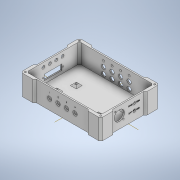
# Autodesk Inventor part: Case
Saved by Autodesk Inventor 2021.1 (Build 251245000, 245)
## iProperties
Created: 2020-06-02
Part Number: Case
Material: Generic
Document SubType Name: Modeling
Designer: Alex
Density: 1 g/cm^3
Appearance: Default
Author: Alex
Autodesk Inventor part; units mm, degrees
note: some values were not read from the file. Chosen so that the rebuilt part matches the saved one: direction of "Hole1"; direction of "Hole2"; direction of "Hole4"; direction of "Hole6"; direction of "Hole7".
(part 1 of 2)
ref_plane "YZ Plane" through (0, 0, 0) normal (1, 0, 0) x (0, 1, 0)
ref_plane "XZ Plane" through (0, 0, 0) normal (0, 1, 0) x (-1, 0, 0)
ref_plane "XY Plane" through (0, 0, 0) normal (0, 0, 1) x (1, 0, 0)
sketch "Sketch1" plane through (0, 0, 0) normal (0, 1, 0) x (-1, 0, 0)
  line L0 (61, -65) -> (-61, -65)
  line L1 (-61, -65) -> (-65, -69)
  line L2 (-65, -69) -> (-90, -69)
  line L3 (-90, -69) -> (-94, -65)
  line L4 (-94, -65) -> (-94, -40)
  line L5 (-94, -40) -> (-90, -36)
  line L6 (-90, -36) -> (-90, 36)
  line L7 (-90, 36) -> (-94, 40)
  line L8 (-94, 40) -> (-94, 65)
  line L9 (-94, 65) -> (-90, 69)
  line L10 (-90, 69) -> (-65, 69)
  line L11 (-65, 69) -> (-61, 65)
  line L12 (-61, 65) -> (61, 65)
  line L13 (61, 65) -> (65, 69)
  line L14 (65, 69) -> (90, 69)
  line L15 (90, 69) -> (94, 65)
  line L16 (94, 65) -> (94, 40)
  line L17 (94, 40) -> (90, 36)
  line L18 (90, 36) -> (90, -36)
  line L19 (90, -36) -> (94, -40)
  line L20 (94, -40) -> (94, -65)
  line L21 (94, -65) -> (90, -69)
  line L22 (90, -69) -> (65, -69)
  line L23 (65, -69) -> (61, -65)
  point P0 (0, 0)
  point P1 (0, -65)
  point P2 (0, 65)
  point P3 (90, 0)
  point P4 (-90, 0)
  dimension "d0" = 135
  dimension "d1" = 130
  dimension "d2" = 180
  dimension "d3" = 4
  dimension "d4" = 25
  constraints: 48 end point, 9 equal length, 9 parallel, 9 perpendicular, 6 point on line, 4 midpoint, 3 collinear, 3 horizontal alignment, 3 vertical alignment, 1 horizontal
  measures "d0" angle of L0 L23
  measures "d1" distance between parallel lines of L12 L0
  measures "d2" distance between parallel lines of L6 L18
  measures "d3" distance between parallel lines of L0 L2
  measures "d4" distance of L1.end L2.end
extrude "Extrusion1" add sketch "Sketch1" along normal blind 3
sketch "Sketch2" plane through (0, 3, 0) normal (0, 1, 0) x (1, 0, 0)
  line L0 (94, 65) -> (90, 69) projected
  line L1 (90, 69) -> (65, 69) projected
  line L2 (65, 69) -> (61, 65) projected
  line L3 (61, 65) -> (-61, 65) projected
  line L4 (-61, 65) -> (-65, 69) projected
  line L5 (-65, 69) -> (-90, 69) projected
  line L6 (-90, 69) -> (-94, 65) projected
  line L7 (-94, 65) -> (-94, 40) projected
  line L8 (-94, 40) -> (-90, 36) projected
  line L9 (-90, 36) -> (-90, -36) projected
  line L10 (-90, -36) -> (-94, -40) projected
  line L11 (-94, -40) -> (-94, -65) projected
  line L12 (-94, -65) -> (-90, -69) projected
  line L13 (-90, -69) -> (-65, -69) projected
  line L14 (-65, -69) -> (-61, -65) projected
  line L15 (-61, -65) -> (61, -65) projected
  line L16 (61, -65) -> (65, -69) projected
  line L17 (65, -69) -> (90, -69) projected
  line L18 (90, -69) -> (94, -65) projected
  line L19 (94, -65) -> (94, -40) projected
  line L20 (94, -40) -> (90, -36) projected
  line L21 (90, -36) -> (90, 36) projected
  line L22 (90, 36) -> (94, 40) projected
  line L23 (94, 40) -> (94, 65) projected
  line L24 (-62.2426, 62) -> (62.2426, 62)
  line L25 (62.2426, 62) -> (66.2426, 66) construction
  line L26 (66.2426, 66) -> (88.7574, 66) construction
  line L27 (88.7574, 66) -> (91, 63.7574) construction
  line L28 (91, 63.7574) -> (91, 41.2426) construction
  line L29 (91, 41.2426) -> (87, 37.2426) construction
  line L30 (87, 37.2426) -> (87, -37.2426)
  line L31 (87, -37.2426) -> (91, -41.2426) construction
  line L32 (91, -41.2426) -> (91, -63.7574) construction
  line L33 (91, -63.7574) -> (88.7574, -66) construction
  line L34 (88.7574, -66) -> (66.2426, -66) construction
  line L35 (66.2426, -66) -> (62.2426, -62) construction
  line L36 (62.2426, -62) -> (-62.2426, -62)
  line L37 (-62.2426, -62) -> (-66.2426, -66) construction
  line L38 (-66.2426, -66) -> (-88.7574, -66) construction
  line L39 (-88.7574, -66) -> (-91, -63.7574) construction
  line L40 (-91, -63.7574) -> (-91, -41.2426) construction
  line L41 (-91, -41.2426) -> (-87, -37.2426) construction
  line L42 (-87, -37.2426) -> (-87, 37.2426)
  line L43 (-87, 37.2426) -> (-91, 41.2426) construction
  line L44 (-91, 41.2426) -> (-91, 63.7574) construction
  line L45 (-91, 63.7574) -> (-88.7574, 66) construction
  line L46 (-88.7574, 66) -> (-66.2426, 66) construction
  line L47 (-66.2426, 66) -> (-62.2426, 62) construction
  line L48 (-62.2426, 62) -> (-83, 62)
  line L49 (-87, 58) -> (-87, 37.2426)
  line L50 (-87, -37.2426) -> (-87, -58)
  line L51 (-83, -62) -> (-62.2426, -62)
  line L52 (62.2426, -62) -> (83, -62)
  line L53 (87, -58) -> (87, -37.2426)
  line L54 (62.2426, 62) -> (83, 62)
  line L55 (87, 58) -> (87, 37.2426)
  line L56 (-87, 58) -> (-83, 62)
  line L57 (-87, -58) -> (-83, -62)
  line L58 (83, -62) -> (87, -58)
  line L59 (87, 58) -> (83, 62)
  point P0 (0, 0)
  point P1 (-87, 62)
  point P2 (-87, -62)
  point P3 (87, -62)
  point P4 (87, 62)
  dimension "d7" = 3
  dimension "d8" = 4
  dimension "d9" = 4
  dimension "d10" = 4
  dimension "d11" = 4
  dimension "d12" = 4
  dimension "d13" = 4
  dimension "d14" = 4
  dimension "d15" = 4
  constraints: 72 end point, 9 point on line, 4 horizontal, 2 perpendicular, 1 vertical, 23 other
  measures "d7" distance between parallel lines of L3 L24
  measures "d8" distance of L49.start point (-87, 62)
  measures "d9" distance of L48.end point (-87, 62)
  measures "d10" distance of L50.end point (-87, -62)
  measures "d11" distance of L51.start point (-87, -62)
  measures "d12" distance of L52.end point (87, -62)
  measures "d13" distance of L53.start point (87, -62)
  measures "d14" distance of L55.start point (87, 62)
  measures "d15" distance of L54.end point (87, 62)
extrude "Extrusion2" add sketch "Sketch2" along normal blind 45
sketch "Sketch3" plane through (0, 3, 0) normal (0, 1, 0) x (1, 0, 0)
  line L0 (60.58, -23.875) -> (-60.58, -23.875) construction
  line L1 (-60.58, -23.875) -> (-60.58, 23.875) construction
  line L2 (-60.58, 23.875) -> (60.58, 23.875) construction
  line L3 (60.58, 23.875) -> (60.58, -23.875) construction
  line L4 (60.58, -23.875) -> (-60.58, 23.875) construction
  line L5 (-60.58, -23.875) -> (60.58, 23.875) construction
  line L6 (-49.356, 16.969) -> (-43.356, 16.969)
  line L7 (-43.356, 16.969) -> (-43.356, 10.969)
  line L8 (-43.356, 10.969) -> (-49.356, 10.969)
  line L9 (-49.356, 10.969) -> (-49.356, 16.969)
  line L10 (-49.356, 16.969) -> (-43.356, 10.969) construction
  line L11 (-43.356, 16.969) -> (-49.356, 10.969) construction
  line L12 (-60.278, -23.575) -> (-54.278, -23.575)
  line L13 (-54.278, -23.575) -> (-54.278, -17.575)
  line L14 (-54.278, -17.575) -> (-60.278, -17.575)
  line L15 (-60.278, -17.575) -> (-60.278, -23.575)
  line L16 (-60.278, -23.575) -> (-54.278, -17.575) construction
  line L17 (-54.278, -23.575) -> (-60.278, -17.575) construction
  line L18 (37.004, -17.575) -> (43.004, -17.575)
  line L19 (43.004, -17.575) -> (43.004, -23.575)
  line L20 (43.004, -23.575) -> (37.004, -23.575)
  line L21 (37.004, -23.575) -> (37.004, -17.575)
  line L22 (37.004, -17.575) -> (43.004, -23.575) construction
  line L23 (43.004, -17.575) -> (37.004, -23.575) construction
  line L24 (54.276, 23.573) -> (60.276, 23.573)
  line L25 (60.276, 23.573) -> (60.276, 17.573)
  line L26 (60.276, 17.573) -> (54.276, 17.573)
  line L27 (54.276, 17.573) -> (54.276, 23.573)
  line L28 (54.276, 23.573) -> (60.276, 17.573) construction
  line L29 (60.276, 23.573) -> (54.276, 17.573) construction
  point P0 (0, 0)
  point P1 (-46.356, 13.969)
  point P2 (-57.278, -20.575)
  point P3 (40.004, -20.575)
  point P4 (57.276, 20.573)
  dimension "d18" = 121.16
  dimension "d19" = 47.75
  dimension "d20" = 9.906
  dimension "d21" = 14.224
  dimension "d28" = 6
  dimension "d188" = 3.302
  dimension "d189" = 44.45
  dimension "d190" = 117.856
  dimension "d191" = 3.302
  dimension "d192" = 100.584
  dimension "d193" = 44.45
  constraints: 60 end point, 10 midpoint, 10 parallel, 6 equal length, 5 horizontal, 5 perpendicular, 1 point on line
  measures "d18" distance of L1.end L2.end
  measures "d19" distance of L2.end L0.start
  measures "d20" distance from line of point (-46.356, 13.969) L2
  measures "d21" distance from line of point (-46.356, 13.969) L1
  measures "d28" distance of L6.end L7.end
  measures "d188" distance from line of point (-57.278, -20.575) L1
  measures "d189" distance from line of point (-57.278, -20.575) L2
  measures "d190" distance from line of point (57.276, 20.573) L1
  measures "d191" distance from line of point (57.276, 20.573) L2
  measures "d192" distance from line of point (40.004, -20.575) L1
  measures "d193" distance from line of point (40.004, -20.575) L2
extrude "Extrusion3" add sketch "Sketch3" along normal blind 4
chamfer "Chamfer1" distance 4 angle 45 16 edges at (40.004, 3, 23.575) (43.004, 3, 20.575) (57.276, 3, -17.573) (60.276, 3, -20.573) (37.004, 3, 20.575) (54.276, 3, -20.573) (40.004, 3, 17.575) (57.276, 3, -23.573) (-57.278, 3, 17.575) (-60.278, 3, 20.575) (-46.356, 3, -16.969) (-49.356, 3, -13.969) (-57.278, 3, 23.575) (-54.278, 3, 20.575) (-46.356, 3, -10.969) (-43.356, 3, -13.969)
sketch "Sketch4" plane through (-61, 0, 65) normal (0, 0, 1) x (1, 0, 0)
  line L0 (0, 0) -> (122, 0) construction
  line L1 (122, 0) -> (122, 48) construction
  line L2 (0, 48) -> (122, 48) construction
  line L3 (0, 0) -> (0, 48) construction
  line L4 (0, 0) -> (0, 48) construction
  line L5 (0, 48) -> (122, 48) construction
  line L6 (61, 48) -> (61, 0) construction
  point P0 (31, 24)
  point P1 (51, 24)
  point P2 (71, 24)
  point P3 (91, 24)
  point P4 (0, 24)
  point P5 (0, 24)
  dimension "d36" = 20
  constraints: 3 midpoint, 2 end point, 1 horizontal, 1 horizontal alignment, 1 perpendicular, 1 symmetric about line, 3 other
  measures "d36" distance of point (31, 24) point (51, 24)
hole "Hole1" at (-30, 24, 65) at (-10, 24, 65) at (10, 24, 65) at (30, 24, 65) direction (0, 0, -1) diameter 10.317 depth 3 clearance for "Hex Head Bolt" size "3/8" standard "Ansi Unified Screw Threads"
sketch "Sketch5" plane through (61, 0, -65) normal (0, 0, -1) x (-1, 0, 0)
  line L0 (0, 0) -> (122, 0) construction
  line L1 (122, 0) -> (122, 48) construction
  line L2 (0, 48) -> (122, 48) construction
  line L3 (0, 0) -> (0, 48) construction
  line L4 (0, 0) -> (0, 48) construction
  line L5 (122, 48) -> (0, 48) construction
  line L6 (61, 48) -> (61, 0) construction
  point P0 (31, 10)
  point P1 (51, 10)
  point P2 (71, 10)
  point P3 (91, 10)
  point P4 (31, 25)
  point P5 (51, 25)
  point P6 (71, 25)
  point P7 (91, 25)
  dimension "d50" = 20
  dimension "d53" = 15
  dimension "d115" = 10
  constraints: 2 end point, 2 vertical, 1 horizontal, 1 midpoint, 1 symmetric about line, 7 other
  measures "d50" distance of point (31, 10) point (51, 10)
  measures "d53" distance of point (31, 10) point (31, 25)
  measures "d115" distance from line of L0 point (31, 10)
hole "Hole2" at (30, 10, -65) at (10, 10, -65) at (-10, 10, -65) at (-30, 10, -65) at (30, 25, -65) at (10, 25, -65) at (-10, 25, -65) at (-30, 25, -65) direction (0, 0, 1) diameter 10.317 depth 3 clearance for "Hex Head Bolt" size "3/8" standard "Ansi Unified Screw Threads"
sketch "Sketch6" plane through (0, 7, 0) normal (0, 1, 0) x (1, 0, 0)
  line L0 (43.004, -17.575) -> (37.004, -17.575) construction
  line L1 (37.004, -17.575) -> (37.004, -23.575) construction
  line L2 (37.004, -23.575) -> (43.004, -23.575) construction
  line L3 (43.004, -23.575) -> (43.004, -17.575) construction
  line L4 (60.276, 23.573) -> (54.276, 23.573) construction
  line L5 (54.276, 23.573) -> (54.276, 17.573) construction
  line L6 (54.276, 17.573) -> (60.276, 17.573) construction
  line L7 (60.276, 17.573) -> (60.276, 23.573) construction
  line L8 (-49.356, 10.969) -> (-43.356, 10.969) construction
  line L9 (-43.356, 10.969) -> (-43.356, 16.969) construction
  line L10 (-43.356, 16.969) -> (-49.356, 16.969) construction
  line L11 (-49.356, 16.969) -> (-49.356, 10.969) construction
  line L12 (-60.278, -17.575) -> (-60.278, -23.575) construction
  line L13 (-60.278, -23.575) -> (-54.278, -23.575) construction
  line L14 (-54.278, -23.575) -> (-54.278, -17.575) construction
  line L15 (-54.278, -17.575) -> (-60.278, -17.575) construction
  point P0 (0, 0)
  point P1 (40.004, -20.575)
  point P2 (57.276, 20.573)
  point P3 (-46.356, 13.969)
  point P4 (-57.278, -20.575)
  point P5 (37.004, -20.575)
  point P6 (-60.278, -20.575)
  point P7 (-49.356, 13.969)
  point P8 (54.276, 20.573)
  point P9 (40.004, -17.575)
  point P10 (57.276, 23.573)
  point P11 (-46.356, 16.969)
  point P12 (-57.278, -17.575)
  constraints: 8 midpoint, 4 horizontal alignment, 4 vertical alignment
hole "Hole3" at (40.004, 7, 20.575) at (57.276, 7, -20.573) at (-46.356, 7, -13.969) at (-57.278, 7, 20.575) direction (0, -1, 0) diameter 4 depth 5
sketch "Sketch7" plane through (-90, 0, -36) normal (-1, 0, 0) x (0, 0, 1)
  line L0 (57, 10) -> (15, 10)
  line L1 (15, 10) -> (15, 23)
  line L2 (15, 23) -> (57, 23)
  line L3 (57, 23) -> (57, 10)
  line L4 (57, 10) -> (15, 23) construction
  line L5 (15, 10) -> (57, 23) construction
  line L6 (0, 0) -> (72, 0) construction
  line L7 (72, 0) -> (72, 48) construction
  line L8 (0, 48) -> (72, 48) construction
  line L9 (0, 0) -> (0, 48) construction
  point P0 (36, 0)
  point P1 (36, 16.5)
  point P2 (36, 48)
  point P3 (36, 16.5)
  point P4 (15, 16.5)
  point P5 (0, 24)
  dimension "d70" = 42
  dimension "d71" = 13
  dimension "d131" = 10
  constraints: 12 end point, 6 midpoint, 2 parallel, 1 horizontal, 1 perpendicular, 1 vertical alignment
  measures "d70" distance of L1.end L2.end
  measures "d71" distance of L2.end L0.start
  measures "d131" distance between parallel lines of L6 L0
extrude "Extrusion4" cut sketch "Sketch7" against normal up to surface (3 mm away)
sketch "Sketch8" plane through (-90, 0, -36) normal (-1, 0, 0) x (0, 0, 1)
  line L0 (9.5, 23) -> (62.5, 23) construction
  line L1 (62.5, 23) -> (62.5, 10) construction
  line L2 (62.5, 10) -> (9.5, 10) construction
  line L3 (9.5, 10) -> (9.5, 23) construction
  line L4 (15, 23) -> (57, 23) construction
  line L5 (57, 23) -> (57, 10) construction
  line L6 (57, 10) -> (15, 10) construction
  line L7 (15, 10) -> (15, 23) construction
  line L8 (0, 0) -> (72, 0) construction
  line L9 (72, 0) -> (72, 48) construction
  line L10 (0, 48) -> (72, 48) construction
  line L11 (0, 0) -> (0, 48) construction
  point P0 (36, 0)
  point P1 (36, 23)
  point P2 (36, 23)
  point P3 (15, 16.5)
  point P4 (9.5, 16.5)
  point P5 (12.5, 16.5)
  point P6 (59.5, 16.5)
  point P7 (57, 16.5)
  dimension "d75" = 53
  dimension "d76" = 3
  dimension "d77" = 3
  constraints: 8 end point, 5 midpoint, 3 horizontal alignment, 2 parallel, 1 coincident, 1 collinear, 1 horizontal, 1 perpendicular
  measures "d75" distance between parallel lines of L3 L1
  measures "d76" distance from line of L3 point (12.5, 16.5)
  measures "d77" distance from line of L1 point (59.5, 16.5)
hole "Hole4" at (-90, 16.5, -23.5) at (-90, 16.5, 23.5) direction (1, 0, 0) diameter 3 depth 3
sketch "Sketch9" plane through (90, 0, 36) normal (1, 0, 0) x (0, 0, -1)
  circle A0 centre (15, 27.5) radius 12
  circle A1 centre (5.5, 39.5) radius 1.75
  circle A2 centre (24.5, 15.5) radius 1.75
  line L0 (28, 12) -> (2, 12) construction
  line L1 (2, 12) -> (2, 43) construction
  line L2 (2, 43) -> (28, 43) construction
  line L3 (28, 43) -> (28, 12) construction
  line L4 (28, 12) -> (2, 43) construction
  line L5 (2, 12) -> (28, 43) construction
  line L6 (0, 0) -> (72, 0) construction
  line L7 (72, 0) -> (72, 48) construction
  line L8 (0, 48) -> (72, 48) construction
  line L9 (0, 0) -> (0, 48) construction
  circle A3 centre (50, 35) radius 3.25
  circle A4 centre (50, 20) radius 3.25
  line L10 (28, 43) -> (72, 43) construction
  line L11 (50, 35) -> (50, 20) construction
  point P0 (36, 0)
  point P1 (2, 27.5)
  point P2 (0, 24)
  point P3 (50, 43)
  point P4 (28, 27.5)
  point P5 (50, 27.5)
  dimension "d85" = 19
  dimension "d86" = 24
  dimension "d87" = 24
  dimension "d88" = 9.5
  dimension "d89" = 12
  dimension "d90" = 3.5
  dimension "d91" = 26
  dimension "d92" = 31
  dimension "d93" = 2
  dimension "d94" = 6.5
  dimension "d95" = 15
  dimension "d194" = 5
  constraints: 16 end point, 7 midpoint, 5 centre point, 2 equal radius, 2 parallel, 2 perpendicular, 2 vertical alignment, 1 horizontal, 1 horizontal alignment, 1 point on line, 1 vertical
  measures "d85" horizontal distance of A2.centre A1.centre
  measures "d86" vertical distance of A2.centre A1.centre
  measures "d87" diameter of A0
  measures "d88" horizontal distance of A0.centre A1.centre
  measures "d89" vertical distance of A0.centre A1.centre
  measures "d90" diameter of A1
  measures "d91" distance of L1.end L2.end
  measures "d92" distance of L2.end L0.start
  measures "d93" distance between parallel lines of L9 L1
  measures "d94" diameter of A3
  measures "d95" distance of L11.start L11.end
  measures "d194" distance between parallel lines of L2 L8
extrude "Extrusion5" cut sketch "Sketch9" against normal up to surface (3 mm away)
sketch "Sketch11" plane through (61, 0, -65) normal (0, 0, -1) x (-1, 0, 0)
  line L0 (-4, 0) -> (0, 0) construction
  line L1 (0, 0) -> (0, 48) construction
  line L2 (-4, 48) -> (0, 48) construction
  line L3 (-4, 0) -> (-4, 48) construction
  circle A0 centre (71, 25) radius 5.1585 construction
  circle A1 centre (31, 25) radius 5.1585 construction
  circle A2 centre (71, 10) radius 5.1585 construction
  circle A3 centre (31, 10) radius 5.1585 construction
  circle A4 centre (51, 10) radius 5.1585 construction
  circle A5 centre (91, 10) radius 5.1585 construction
  circle A6 centre (51, 25) radius 5.1585 construction
  circle A7 centre (91, 25) radius 5.1585 construction
  line L4 (0, 0) -> (122, 0) construction
  line L5 (122, 0) -> (122, 48) construction
  line L6 (0, 48) -> (122, 48) construction
  line L7 (0, 0) -> (0, 48) construction
  point P0 (61, 0)
  point P1 (31, 37.5)
  point P2 (51, 37.5)
  point P3 (71, 37.5)
  point P4 (91, 37.5)
  dimension "d118" = 20
  dimension "d147" = 12.5
  constraints: 1 horizontal, 1 vertical alignment, 3 other
  measures "d118" distance of point (31, 37.5) point (51, 37.5)
  measures "d147" distance of A1.centre point (31, 37.5)
hole "Hole6" at (30, 37.5, -65) at (10, 37.5, -65) at (-10, 37.5, -65) at (-30, 37.5, -65) direction (0, 0, 1) diameter 5 depth 3
sketch "Sketch12" plane through (-90, 0, -36) normal (-1, 0, 0) x (0, 0, 1)
  circle A0 centre (12.5, 16.5) radius 1.5 construction
  circle A1 centre (59.5, 16.5) radius 1.5 construction
  line L0 (15, 10) -> (15, 23) construction
  line L1 (15, 23) -> (57, 23) construction
  line L2 (57, 23) -> (57, 10) construction
  line L3 (57, 10) -> (15, 10) construction
  line L4 (0, 0) -> (72, 0) construction
  line L5 (72, 0) -> (72, 48) construction
  line L6 (0, 48) -> (72, 48) construction
  line L7 (0, 0) -> (0, 48) construction
  line L8 (-22, 48) -> (94, 48) construction
  line L9 (36, 48) -> (36, 0) construction
  line L10 (72, 0) -> (0, 0) construction
  point P0 (13.5, 38)
  point P1 (28.5, 38)
  point P2 (43.5, 38)
  point P3 (58.5, 38)
  dimension "d134" = 15
  dimension "d139" = 10
  constraints: 2 end point, 1 horizontal, 1 midpoint, 1 perpendicular, 1 symmetric about line, 3 other
  measures "d134" distance of point (13.5, 38) point (28.5, 38)
  measures "d139" distance from line of point (28.5, 38) L6
hole "Hole7" at (-90, 38, -22.5) at (-90, 38, -7.5) at (-90, 38, 7.5) at (-90, 38, 22.5) direction (1, 0, 0) diameter 7 depth 3
sketch "Sketch13" plane through (-61, 0, 65) normal (0, 0, 1) x (1, 0, 0)
  line L0 (28.5, 39) -> (33.5, 39) construction
  line L1 (33.5, 39) -> (33.5, 34) construction
  line L2 (33.5, 34) -> (28.5, 34) construction
  line L3 (28.5, 34) -> (28.5, 39) construction
  line L4 (48.5, 39) -> (53.5, 39) construction
  line L5 (53.5, 39) -> (53.5, 34) construction
  line L6 (53.5, 34) -> (48.5, 34) construction
  line L7 (48.5, 34) -> (48.5, 39) construction
  line L8 (68.5, 39) -> (73.5, 39) construction
  line L9 (73.5, 39) -> (73.5, 34) construction
  line L10 (73.5, 34) -> (68.5, 34) construction
  line L11 (68.5, 34) -> (68.5, 39) construction
  line L12 (88.5, 39) -> (93.5, 39) construction
  line L13 (93.5, 39) -> (93.5, 34) construction
  line L14 (93.5, 34) -> (88.5, 34) construction
  line L15 (88.5, 34) -> (88.5, 39) construction
  circle A0 centre (71, 24) radius 5.1585 construction
  circle A1 centre (31, 24) radius 5.1585 construction
  circle A2 centre (51, 24) radius 5.1585 construction
  circle A3 centre (91, 24) radius 5.1585 construction
  line L16 (0, 0) -> (122, 0) construction
  line L17 (122, 0) -> (122, 48) construction
  line L18 (0, 48) -> (122, 48) construction
  line L19 (0, 0) -> (0, 48) construction
  spline S0 degree 2 poles (31.0949, 35.1624) (31.0949, 34.9797) (30.9145, 34.9797) knots 0 0 0 1 1 1
  spline S1 degree 2 poles (30.9145, 34.9797) (30.7318, 34.9797) (30.7318, 35.1624) knots 0 0 0 1 1 1
  line L20 (30.7318, 35.1624) -> (30.7318, 37.8376)
  spline S2 degree 2 poles (30.7318, 37.8376) (30.7318, 38.0203) (30.9145, 38.0203) knots 0 0 0 1 1 1
  spline S3 degree 2 poles (30.9145, 38.0203) (31.0949, 38.0203) (31.0949, 37.8376) knots 0 0 0 1 1 1
  line L21 (31.0949, 37.8376) -> (31.0949, 35.1624)
  line L22 (51.6313, 34.9855) -> (49.9915, 34.9855)
  spline S4 degree 2 poles (49.9915, 34.9855) (50.0665, 35.2924) (50.1415, 35.5923) knots 0 0 0 1 1 1
  spline S5 degree 2 poles (50.1415, 35.5923) (50.2562, 35.9647) (50.4647, 36.2411) knots 0 0 0 1 1 1
  spline S6 degree 2 poles (50.4647, 36.2411) (50.7318, 36.5902) (51.2097, 36.8666) knots 0 0 0 1 1 1
  spline S7 degree 2 poles (51.2097, 36.8666) (51.458, 37.0072) (51.458, 37.2602) knots 0 0 0 1 1 1
  spline S8 degree 2 poles (51.458, 37.2602) (51.458, 37.4195) (51.2354, 37.642) (51.0504, 37.642) knots 0 0 0 1 2 2 2
  spline S9 degree 2 poles (51.0504, 37.642) (50.8278, 37.642) (50.7084, 37.5717) knots 0 0 0 1 1 1
  spline S10 degree 2 poles (50.7084, 37.5717) (50.5678, 37.4921) (50.4835, 37.2789) knots 0 0 0 1 1 1
  spline S11 degree 2 poles (50.4835, 37.2789) (50.439, 37.1665) (50.3335, 37.1665) knots 0 0 0 1 1 1
  spline S12 degree 2 poles (50.3335, 37.1665) (50.2609, 37.1665) (50.1508, 37.2695) (50.1508, 37.3445) knots 0 0 0 1 2 2 2
  spline S13 degree 2 poles (50.1508, 37.3445) (50.1508, 37.3843) (50.1696, 37.4241) knots 0 0 0 1 1 1
  spline S14 degree 2 poles (50.1696, 37.4241) (50.3991, 38.0145) (51.034, 38.0145) knots 0 0 0 1 1 1
  spline S15 degree 2 poles (51.034, 38.0145) (51.4111, 38.0145) (51.636, 37.7966) knots 0 0 0 1 1 1
  spline S16 degree 2 poles (51.636, 37.7966) (51.8445, 37.5928) (51.8445, 37.2906) knots 0 0 0 1 1 1
  spline S17 degree 2 poles (51.8445, 37.2906) (51.8445, 36.8174) (50.9145, 36.2669) (50.692, 35.9202) knots 0 0 0 1 2 2 2
  spline S18 degree 2 poles (50.692, 35.9202) (50.5537, 35.7094) (50.4671, 35.358) knots 0 0 0 1 1 1
  line L23 (50.4671, 35.358) -> (51.6313, 35.358)
  spline S19 degree 2 poles (51.6313, 35.358) (51.814, 35.358) (51.814, 35.1729) knots 0 0 0 1 1 1
  spline S20 degree 2 poles (51.814, 35.1729) (51.814, 34.9855) (51.6313, 34.9855) knots 0 0 0 1 1 1
  spline S21 degree 2 poles (71.8281, 36.0783) (71.8281, 35.5677) (71.5259, 35.2561) knots 0 0 0 1 1 1
  spline S22 degree 2 poles (71.5259, 35.2561) (71.2518, 34.9773) (70.863, 34.9773) knots 0 0 0 1 1 1
  spline S23 degree 2 poles (70.863, 34.9773) (70.5608, 34.9773) (70.3218, 35.1554) knots 0 0 0 1 1 1
  spline S24 degree 2 poles (70.3218, 35.1554) (70.0595, 35.3498) (69.9494, 35.7012) knots 0 0 0 1 1 1
  spline S25 degree 2 poles (69.9494, 35.7012) (69.94, 35.7316) (69.94, 35.7621) knots 0 0 0 1 1 1
  spline S26 degree 2 poles (69.94, 35.7621) (69.94, 35.8417) (70.0501, 35.9401) (70.1227, 35.9401) knots 0 0 0 1 2 2 2
  spline S27 degree 2 poles (70.1227, 35.9401) (70.2469, 35.9401) (70.2867, 35.816) knots 0 0 0 1 1 1
  spline S28 degree 2 poles (70.2867, 35.816) (70.3523, 35.5981) (70.5163, 35.474) knots 0 0 0 1 1 1
  spline S29 degree 2 poles (70.5163, 35.474) (70.6662, 35.3639) (70.8536, 35.3639) knots 0 0 0 1 1 1
  spline S30 degree 2 poles (70.8536, 35.3639) (71.1019, 35.3639) (71.2799, 35.5489) knots 0 0 0 1 1 1
  spline S31 degree 2 poles (71.2799, 35.5489) (71.4744, 35.7504) (71.4744, 36.0783) knots 0 0 0 1 1 1
  spline S32 degree 2 poles (71.4744, 36.0783) (71.4744, 36.4274) (71.2706, 36.6101) knots 0 0 0 1 1 1
  spline S33 degree 2 poles (71.2706, 36.6101) (71.1206, 36.7366) (70.8676, 36.7764) knots 0 0 0 1 1 1
  spline S34 degree 2 poles (70.8676, 36.7764) (70.7341, 36.7858) (70.5959, 36.7952) knots 0 0 0 1 1 1
  spline S35 degree 2 poles (70.5959, 36.7952) (70.5209, 36.7998) (70.4226, 36.8935) (70.4226, 36.9404) knots 0 0 0 1 2 2 2
  spline S36 degree 2 poles (70.4226, 36.9404) (70.4226, 37.0294) (70.4999, 37.1091) knots 0 0 0 1 1 1
  line L24 (70.4999, 37.1091) -> (71.0129, 37.6502)
  line L25 (71.0129, 37.6502) -> (70.2469, 37.6502)
  spline S37 degree 2 poles (70.2469, 37.6502) (70.0688, 37.6502) (70.0688, 37.8329) knots 0 0 0 1 1 1
  spline S38 degree 2 poles (70.0688, 37.8329) (70.0688, 38.018) (70.2469, 38.018) knots 0 0 0 1 1 1
  line L26 (70.2469, 38.018) -> (71.5892, 38.0227)
  spline S39 degree 2 poles (71.5892, 38.0227) (71.7133, 38.0227) (71.7133, 37.9313) knots 0 0 0 1 1 1
  spline S40 degree 2 poles (71.7133, 37.9313) (71.7133, 37.8634) (71.5517, 37.697) knots 0 0 0 1 1 1
  line L27 (71.5517, 37.697) -> (71.0269, 37.1372)
  spline S41 degree 2 poles (71.0269, 37.1372) (71.8281, 36.9779) (71.8281, 36.0783) knots 0 0 0 1 1 1
  line L28 (91.807, 35.4505) -> (91.5634, 35.4505)
  line L29 (91.5634, 35.4505) -> (91.5634, 35.1624)
  spline S42 degree 2 poles (91.5634, 35.1624) (91.5634, 34.975) (91.383, 34.975) knots 0 0 0 1 1 1
  spline S43 degree 2 poles (91.383, 34.975) (91.2003, 34.975) (91.2003, 35.1624) knots 0 0 0 1 1 1
  line L30 (91.2003, 35.1624) -> (91.2003, 35.4505)
  line L31 (91.2003, 35.4505) -> (89.9236, 35.4505)
  spline S44 degree 2 poles (89.9236, 35.4505) (89.7994, 35.4505) (89.7994, 35.645) knots 0 0 0 1 1 1
  spline S45 degree 2 poles (89.7994, 35.645) (89.7994, 35.7293) (89.8252, 35.8089) knots 0 0 0 1 1 1
  line L32 (89.8252, 35.8089) -> (90.5537, 37.9008)
  spline S46 degree 2 poles (90.5537, 37.9008) (90.5983, 38.025) (90.7177, 38.025) knots 0 0 0 1 1 1
  spline S47 degree 2 poles (90.7177, 38.025) (90.7927, 38.025) (90.9168, 37.9196) (90.9168, 37.8446) knots 0 0 0 1 2 2 2
  spline S48 degree 2 poles (90.9168, 37.8446) (90.9168, 37.8071) (90.9051, 37.7767) knots 0 0 0 1 1 1
  line L33 (90.9051, 37.7767) -> (90.2352, 35.823)
  line L34 (90.2352, 35.823) -> (91.2003, 35.823)
  line L35 (91.2003, 35.823) -> (91.2003, 36.336)
  spline S49 degree 2 poles (91.2003, 36.336) (91.2003, 36.5234) (91.383, 36.5234) knots 0 0 0 1 1 1
  spline S50 degree 2 poles (91.383, 36.5234) (91.5634, 36.5234) (91.5634, 36.336) knots 0 0 0 1 1 1
  line L36 (91.5634, 36.336) -> (91.5634, 35.823)
  line L37 (91.5634, 35.823) -> (91.8094, 35.823)
  spline S51 degree 2 poles (91.8094, 35.823) (91.9944, 35.823) (91.9944, 35.6379) knots 0 0 0 1 1 1
  spline S52 degree 2 poles (91.9944, 35.6379) (91.9944, 35.4505) (91.807, 35.4505) knots 0 0 0 1 1 1
  point P0 (61, 0)
  point P1 (31, 34)
  point P2 (51, 34)
  point P3 (71, 34)
  point P4 (91, 34)
  dimension "d148" = 5
  dimension "d149" = 5
  dimension "d150" = 10
  constraints: 6 equal length, 6 horizontal alignment, 4 midpoint, 4 vertical alignment, 2 horizontal, 8 other
  measures "d148" distance of L0.start L0.end
  measures "d149" distance of L2.end L0.start
  measures "d150" distance of A1.centre point (31, 34)
emboss "Emboss1" sketch "Sketch13" operation cut depth 1 direction (0, 0, -1)
sketch "Sketch14" plane through (61, 0, -65) normal (0, 0, -1) x (-1, 0, 0)
  line L0 (28.5, 46.5) -> (33.5, 46.5) construction
  line L1 (33.5, 46.5) -> (33.5, 41.5) construction
  line L2 (33.5, 41.5) -> (28.5, 41.5) construction
  line L3 (28.5, 41.5) -> (28.5, 46.5) construction
  line L4 (88.5, 46.5) -> (93.5, 46.5) construction
  line L5 (93.5, 46.5) -> (93.5, 41.5) construction
  line L6 (93.5, 41.5) -> (88.5, 41.5) construction
  line L7 (88.5, 41.5) -> (88.5, 46.5) construction
  line L8 (68.5, 46.5) -> (73.5, 46.5) construction
  line L9 (73.5, 46.5) -> (73.5, 41.5) construction
  line L10 (73.5, 41.5) -> (68.5, 41.5) construction
  line L11 (68.5, 41.5) -> (68.5, 46.5) construction
  line L12 (48.5, 46.5) -> (53.5, 46.5) construction
  line L13 (53.5, 46.5) -> (53.5, 41.5) construction
  line L14 (53.5, 41.5) -> (48.5, 41.5) construction
  line L15 (48.5, 41.5) -> (48.5, 46.5) construction
  circle A0 centre (71, 37.5) radius 2.5 construction
  circle A1 centre (31, 37.5) radius 2.5 construction
  circle A2 centre (51, 37.5) radius 2.5 construction
  circle A3 centre (91, 37.5) radius 2.5 construction
  circle A4 centre (71, 25) radius 5.1585 construction
  circle A5 centre (31, 25) radius 5.1585 construction
  circle A6 centre (71, 10) radius 5.1585 construction
  circle A7 centre (31, 10) radius 5.1585 construction
  circle A8 centre (51, 10) radius 5.1585 construction
  circle A9 centre (91, 10) radius 5.1585 construction
  circle A10 centre (51, 25) radius 5.1585 construction
  circle A11 centre (91, 25) radius 5.1585 construction
  line L16 (0, 0) -> (122, 0) construction
  line L17 (122, 0) -> (122, 48) construction
  line L18 (0, 48) -> (122, 48) construction
  line L19 (0, 0) -> (0, 48) construction
  line L20 (11, 12.5) -> (16, 12.5) construction
  line L21 (16, 12.5) -> (16, 7.5) construction
  line L22 (16, 7.5) -> (11, 7.5) construction
  line L23 (11, 7.5) -> (11, 12.5) construction
  line L24 (11, 27.5) -> (16, 27.5) construction
  line L25 (16, 27.5) -> (16, 22.5) construction
  line L26 (16, 22.5) -> (11, 22.5) construction
  line L27 (11, 22.5) -> (11, 27.5) construction
  spline S0 degree 2 poles (13.1615, 23.6601) (13.1615, 23.4727) (13.0139, 23.4727) knots 0 0 0 1 1 1
  spline S1 degree 2 poles (13.0139, 23.4727) (12.9015, 23.4727) (12.8125, 23.5992) knots 0 0 0 1 1 1
  line L28 (12.8125, 23.5992) -> (11.3203, 25.7777)
  line L29 (11.3203, 25.7777) -> (11.3203, 23.6624)
  spline S2 degree 2 poles (11.3203, 23.6624) (11.3203, 23.4727) (11.1399, 23.4727) knots 0 0 0 1 1 1
  spline S3 degree 2 poles (11.1399, 23.4727) (10.9572, 23.4727) (10.9572, 23.6624) knots 0 0 0 1 1 1
  line L30 (10.9572, 23.6624) -> (10.9572, 26.3493)
  spline S4 degree 2 poles (10.9572, 26.3493) (10.9572, 26.5273) (11.1211, 26.5273) knots 0 0 0 1 1 1
  spline S5 degree 2 poles (11.1211, 26.5273) (11.2359, 26.5273) (11.3203, 26.4079) knots 0 0 0 1 1 1
  line L31 (11.3203, 26.4079) -> (12.7984, 24.2668)
  line L32 (12.7984, 24.2668) -> (12.7984, 26.3353)
  spline S6 degree 2 poles (12.7984, 26.3353) (12.7984, 26.5273) (12.9811, 26.5273) knots 0 0 0 1 1 1
  spline S7 degree 2 poles (12.9811, 26.5273) (13.1615, 26.5273) (13.1615, 26.3353) knots 0 0 0 1 1 1
  line L33 (13.1615, 26.3353) -> (13.1615, 23.6601)
  spline S8 degree 2 poles (15.8765, 23.9388) (15.6563, 23.6624) (15.2347, 23.4539) (14.9372, 23.4539) knots 0 0 0 1 2 2 2
  spline S9 degree 2 poles (14.9372, 23.4539) (14.4358, 23.4539) (14.1173, 23.8803) knots 0 0 0 1 1 1
  spline S10 degree 2 poles (14.1173, 23.8803) (13.7846, 24.3183) (13.7846, 25.0281) knots 0 0 0 1 1 1
  spline S11 degree 2 poles (13.7846, 25.0281) (13.7846, 25.8152) (14.1571, 26.2228) knots 0 0 0 1 1 1
  spline S12 degree 2 poles (14.1571, 26.2228) (14.4546, 26.5461) (14.8762, 26.5461) knots 0 0 0 1 1 1
  spline S13 degree 2 poles (14.8762, 26.5461) (15.2136, 26.5461) (15.4033, 26.4477) knots 0 0 0 1 1 1
  spline S14 degree 2 poles (15.4033, 26.4477) (15.6118, 26.3423) (15.7617, 26.0659) knots 0 0 0 1 1 1
  spline S15 degree 2 poles (15.7617, 26.0659) (15.7898, 26.019) (15.7898, 25.9745) knots 0 0 0 1 1 1
  spline S16 degree 2 poles (15.7898, 25.9745) (15.7898, 25.8972) (15.6727, 25.7918) (15.6024, 25.7918) knots 0 0 0 1 2 2 2
  spline S17 degree 2 poles (15.6024, 25.7918) (15.5041, 25.7918) (15.4525, 25.8855) knots 0 0 0 1 1 1
  spline S18 degree 2 poles (15.4525, 25.8855) (15.3588, 26.0541) (15.2159, 26.1151) knots 0 0 0 1 1 1
  spline S19 degree 2 poles (15.2159, 26.1151) (15.0918, 26.1736) (14.8739, 26.1736) knots 0 0 0 1 1 1
  spline S20 degree 2 poles (14.8739, 26.1736) (14.5834, 26.1736) (14.382, 25.9159) knots 0 0 0 1 1 1
  spline S21 degree 2 poles (14.382, 25.9159) (14.143, 25.6091) (14.143, 25.0281) knots 0 0 0 1 1 1
  spline S22 degree 2 poles (14.143, 25.0281) (14.143, 24.4964) (14.5951, 23.8264) (14.9465, 23.8264) knots 0 0 0 1 2 2 2
  spline S23 degree 2 poles (14.9465, 23.8264) (15.319, 23.8264) (15.5978, 24.1778) knots 0 0 0 1 1 1
  spline S24 degree 2 poles (15.5978, 24.1778) (15.6516, 24.2434) (15.7313, 24.2434) knots 0 0 0 1 1 1
  spline S25 degree 2 poles (15.7313, 24.2434) (15.8016, 24.2434) (15.921, 24.1286) (15.921, 24.0536) knots 0 0 0 1 2 2 2
  spline S26 degree 2 poles (15.921, 24.0536) (15.921, 23.9904) (15.8765, 23.9388) knots 0 0 0 1 1 1
  spline S27 degree 2 poles (13.1111, 8.6601) (13.1111, 8.4727) (12.9636, 8.4727) knots 0 0 0 1 1 1
  spline S28 degree 2 poles (12.9636, 8.4727) (12.8511, 8.4727) (12.7621, 8.5992) knots 0 0 0 1 1 1
  line L34 (12.7621, 8.5992) -> (11.2699, 10.7777)
  line L35 (11.2699, 10.7777) -> (11.2699, 8.6624)
  spline S29 degree 2 poles (11.2699, 8.6624) (11.2699, 8.4727) (11.0895, 8.4727) knots 0 0 0 1 1 1
  spline S30 degree 2 poles (11.0895, 8.4727) (10.9068, 8.4727) (10.9068, 8.6624) knots 0 0 0 1 1 1
  line L36 (10.9068, 8.6624) -> (10.9068, 11.3493)
  spline S31 degree 2 poles (10.9068, 11.3493) (10.9068, 11.5273) (11.0708, 11.5273) knots 0 0 0 1 1 1
  spline S32 degree 2 poles (11.0708, 11.5273) (11.1856, 11.5273) (11.2699, 11.4079) knots 0 0 0 1 1 1
  line L37 (11.2699, 11.4079) -> (12.748, 9.2668)
  line L38 (12.748, 9.2668) -> (12.748, 11.3353)
  spline S33 degree 2 poles (12.748, 11.3353) (12.748, 11.5273) (12.9308, 11.5273) knots 0 0 0 1 1 1
  spline S34 degree 2 poles (12.9308, 11.5273) (13.1111, 11.5273) (13.1111, 11.3353) knots 0 0 0 1 1 1
  line L39 (13.1111, 11.3353) -> (13.1111, 8.6601)
  spline S35 degree 2 poles (16.0276, 9.9836) (16.0276, 9.3675) (15.7301, 8.9295) knots 0 0 0 1 1 1
  spline S36 degree 2 poles (15.7301, 8.9295) (15.4068, 8.4539) (14.8962, 8.4539) knots 0 0 0 1 1 1
  spline S37 degree 2 poles (14.8962, 8.4539) (14.3878, 8.4539) (14.0599, 8.9295) knots 0 0 0 1 1 1
  spline S38 degree 2 poles (14.0599, 8.9295) (13.7483, 9.3722) (13.7483, 9.9836) knots 0 0 0 1 1 1
  spline S39 degree 2 poles (13.7483, 9.9836) (13.7483, 10.602) (14.0411, 11.0541) knots 0 0 0 1 1 1
  spline S40 degree 2 poles (14.0411, 11.0541) (14.355, 11.5461) (14.847, 11.5461) knots 0 0 0 1 1 1
  spline S41 degree 2 poles (14.847, 11.5461) (15.3764, 11.5461) (15.7161, 11.0541) knots 0 0 0 1 1 1
  spline S42 degree 2 poles (15.7161, 11.0541) (16.0276, 10.602) (16.0276, 9.9836) knots 0 0 0 1 1 1
  spline S43 degree 2 poles (15.6645, 9.9836) (15.6645, 10.4591) (15.4654, 10.7965) knots 0 0 0 1 1 1
  spline S44 degree 2 poles (15.4654, 10.7965) (15.2335, 11.1736) (14.847, 11.1736) knots 0 0 0 1 1 1
  spline S45 degree 2 poles (14.847, 11.1736) (14.4886, 11.1736) (14.2894, 10.7965) knots 0 0 0 1 1 1
  spline S46 degree 2 poles (14.2894, 10.7965) (14.1114, 10.4685) (14.1114, 9.9836) knots 0 0 0 1 1 1
  spline S47 degree 2 poles (14.1114, 9.9836) (14.1114, 9.5151) (14.3058, 9.1895) knots 0 0 0 1 1 1
  spline S48 degree 2 poles (14.3058, 9.1895) (14.5237, 8.8264) (14.8962, 8.8264) knots 0 0 0 1 1 1
  spline S49 degree 2 poles (14.8962, 8.8264) (15.2686, 8.8264) (15.4818, 9.1895) knots 0 0 0 1 1 1
  spline S50 degree 2 poles (15.4818, 9.1895) (15.6645, 9.5104) (15.6645, 9.9836) knots 0 0 0 1 1 1
  line L40 (31.807, 42.9505) -> (31.5634, 42.9505)
  line L41 (31.5634, 42.9505) -> (31.5634, 42.6624)
  spline S51 degree 2 poles (31.5634, 42.6624) (31.5634, 42.475) (31.383, 42.475) knots 0 0 0 1 1 1
  spline S52 degree 2 poles (31.383, 42.475) (31.2003, 42.475) (31.2003, 42.6624) knots 0 0 0 1 1 1
  line L42 (31.2003, 42.6624) -> (31.2003, 42.9505)
  line L43 (31.2003, 42.9505) -> (29.9236, 42.9505)
  spline S53 degree 2 poles (29.9236, 42.9505) (29.7994, 42.9505) (29.7994, 43.145) knots 0 0 0 1 1 1
  spline S54 degree 2 poles (29.7994, 43.145) (29.7994, 43.2293) (29.8252, 43.3089) knots 0 0 0 1 1 1
  line L44 (29.8252, 43.3089) -> (30.5537, 45.4008)
  spline S55 degree 2 poles (30.5537, 45.4008) (30.5983, 45.525) (30.7177, 45.525) knots 0 0 0 1 1 1
  spline S56 degree 2 poles (30.7177, 45.525) (30.7927, 45.525) (30.9168, 45.4196) (30.9168, 45.3446) knots 0 0 0 1 2 2 2
  spline S57 degree 2 poles (30.9168, 45.3446) (30.9168, 45.3071) (30.9051, 45.2767) knots 0 0 0 1 1 1
  line L45 (30.9051, 45.2767) -> (30.2352, 43.323)
  line L46 (30.2352, 43.323) -> (31.2003, 43.323)
  line L47 (31.2003, 43.323) -> (31.2003, 43.836)
  spline S58 degree 2 poles (31.2003, 43.836) (31.2003, 44.0234) (31.383, 44.0234) knots 0 0 0 1 1 1
  spline S59 degree 2 poles (31.383, 44.0234) (31.5634, 44.0234) (31.5634, 43.836) knots 0 0 0 1 1 1
  line L48 (31.5634, 43.836) -> (31.5634, 43.323)
  line L49 (31.5634, 43.323) -> (31.8094, 43.323)
  spline S60 degree 2 poles (31.8094, 43.323) (31.9944, 43.323) (31.9944, 43.1379) knots 0 0 0 1 1 1
  spline S61 degree 2 poles (31.9944, 43.1379) (31.9944, 42.9505) (31.807, 42.9505) knots 0 0 0 1 1 1
  spline S62 degree 2 poles (51.8281, 43.5783) (51.8281, 43.0677) (51.5259, 42.7561) knots 0 0 0 1 1 1
  spline S63 degree 2 poles (51.5259, 42.7561) (51.2518, 42.4773) (50.863, 42.4773) knots 0 0 0 1 1 1
  spline S64 degree 2 poles (50.863, 42.4773) (50.5608, 42.4773) (50.3218, 42.6554) knots 0 0 0 1 1 1
  spline S65 degree 2 poles (50.3218, 42.6554) (50.0595, 42.8498) (49.9494, 43.2012) knots 0 0 0 1 1 1
  spline S66 degree 2 poles (49.9494, 43.2012) (49.94, 43.2316) (49.94, 43.2621) knots 0 0 0 1 1 1
  spline S67 degree 2 poles (49.94, 43.2621) (49.94, 43.3417) (50.0501, 43.4401) (50.1227, 43.4401) knots 0 0 0 1 2 2 2
  spline S68 degree 2 poles (50.1227, 43.4401) (50.2469, 43.4401) (50.2867, 43.316) knots 0 0 0 1 1 1
  spline S69 degree 2 poles (50.2867, 43.316) (50.3523, 43.0981) (50.5163, 42.974) knots 0 0 0 1 1 1
  spline S70 degree 2 poles (50.5163, 42.974) (50.6662, 42.8639) (50.8536, 42.8639) knots 0 0 0 1 1 1
  spline S71 degree 2 poles (50.8536, 42.8639) (51.1019, 42.8639) (51.2799, 43.0489) knots 0 0 0 1 1 1
  spline S72 degree 2 poles (51.2799, 43.0489) (51.4744, 43.2504) (51.4744, 43.5783) knots 0 0 0 1 1 1
  spline S73 degree 2 poles (51.4744, 43.5783) (51.4744, 43.9274) (51.2706, 44.1101) knots 0 0 0 1 1 1
  spline S74 degree 2 poles (51.2706, 44.1101) (51.1206, 44.2366) (50.8676, 44.2764) knots 0 0 0 1 1 1
  spline S75 degree 2 poles (50.8676, 44.2764) (50.7341, 44.2858) (50.5959, 44.2952) knots 0 0 0 1 1 1
  spline S76 degree 2 poles (50.5959, 44.2952) (50.5209, 44.2998) (50.4226, 44.3935) (50.4226, 44.4404) knots 0 0 0 1 2 2 2
  spline S77 degree 2 poles (50.4226, 44.4404) (50.4226, 44.5294) (50.4999, 44.6091) knots 0 0 0 1 1 1
  line L50 (50.4999, 44.6091) -> (51.0129, 45.1502)
  line L51 (51.0129, 45.1502) -> (50.2469, 45.1502)
  spline S78 degree 2 poles (50.2469, 45.1502) (50.0688, 45.1502) (50.0688, 45.3329) knots 0 0 0 1 1 1
  spline S79 degree 2 poles (50.0688, 45.3329) (50.0688, 45.518) (50.2469, 45.518) knots 0 0 0 1 1 1
  line L52 (50.2469, 45.518) -> (51.5892, 45.5227)
  spline S80 degree 2 poles (51.5892, 45.5227) (51.7133, 45.5227) (51.7133, 45.4313) knots 0 0 0 1 1 1
  spline S81 degree 2 poles (51.7133, 45.4313) (51.7133, 45.3634) (51.5517, 45.197) knots 0 0 0 1 1 1
  line L53 (51.5517, 45.197) -> (51.0269, 44.6372)
  spline S82 degree 2 poles (51.0269, 44.6372) (51.8281, 44.4779) (51.8281, 43.5783) knots 0 0 0 1 1 1
  line L54 (71.6313, 42.4855) -> (69.9915, 42.4855)
  spline S83 degree 2 poles (69.9915, 42.4855) (70.0665, 42.7924) (70.1415, 43.0923) knots 0 0 0 1 1 1
  spline S84 degree 2 poles (70.1415, 43.0923) (70.2562, 43.4647) (70.4647, 43.7411) knots 0 0 0 1 1 1
  spline S85 degree 2 poles (70.4647, 43.7411) (70.7318, 44.0902) (71.2097, 44.3666) knots 0 0 0 1 1 1
  spline S86 degree 2 poles (71.2097, 44.3666) (71.458, 44.5072) (71.458, 44.7602) knots 0 0 0 1 1 1
  spline S87 degree 2 poles (71.458, 44.7602) (71.458, 44.9195) (71.2354, 45.142) (71.0504, 45.142) knots 0 0 0 1 2 2 2
  spline S88 degree 2 poles (71.0504, 45.142) (70.8278, 45.142) (70.7084, 45.0717) knots 0 0 0 1 1 1
  spline S89 degree 2 poles (70.7084, 45.0717) (70.5678, 44.9921) (70.4835, 44.7789) knots 0 0 0 1 1 1
  spline S90 degree 2 poles (70.4835, 44.7789) (70.439, 44.6665) (70.3335, 44.6665) knots 0 0 0 1 1 1
  spline S91 degree 2 poles (70.3335, 44.6665) (70.2609, 44.6665) (70.1508, 44.7695) (70.1508, 44.8445) knots 0 0 0 1 2 2 2
  spline S92 degree 2 poles (70.1508, 44.8445) (70.1508, 44.8843) (70.1696, 44.9241) knots 0 0 0 1 1 1
  spline S93 degree 2 poles (70.1696, 44.9241) (70.3991, 45.5145) (71.034, 45.5145) knots 0 0 0 1 1 1
  spline S94 degree 2 poles (71.034, 45.5145) (71.4111, 45.5145) (71.636, 45.2966) knots 0 0 0 1 1 1
  spline S95 degree 2 poles (71.636, 45.2966) (71.8445, 45.0928) (71.8445, 44.7906) knots 0 0 0 1 1 1
  spline S96 degree 2 poles (71.8445, 44.7906) (71.8445, 44.3174) (70.9145, 43.7669) (70.692, 43.4202) knots 0 0 0 1 2 2 2
  spline S97 degree 2 poles (70.692, 43.4202) (70.5537, 43.2094) (70.4671, 42.858) knots 0 0 0 1 1 1
  line L55 (70.4671, 42.858) -> (71.6313, 42.858)
  spline S98 degree 2 poles (71.6313, 42.858) (71.814, 42.858) (71.814, 42.6729) knots 0 0 0 1 1 1
  spline S99 degree 2 poles (71.814, 42.6729) (71.814, 42.4855) (71.6313, 42.4855) knots 0 0 0 1 1 1
  spline S100 degree 2 poles (91.0949, 42.6624) (91.0949, 42.4797) (90.9145, 42.4797) knots 0 0 0 1 1 1
  spline S101 degree 2 poles (90.9145, 42.4797) (90.7318, 42.4797) (90.7318, 42.6624) knots 0 0 0 1 1 1
  line L56 (90.7318, 42.6624) -> (90.7318, 45.3376)
  spline S102 degree 2 poles (90.7318, 45.3376) (90.7318, 45.5203) (90.9145, 45.5203) knots 0 0 0 1 1 1
  spline S103 degree 2 poles (90.9145, 45.5203) (91.0949, 45.5203) (91.0949, 45.3376) knots 0 0 0 1 1 1
  line L57 (91.0949, 45.3376) -> (91.0949, 42.6624)
  point P0 (61, 0)
  point P1 (91, 41.5)
  point P2 (71, 41.5)
  point P3 (51, 41.5)
  point P4 (31, 41.5)
  point P5 (13.5, 7.5)
  point P6 (13.5, 22.5)
  point P7 (16, 25)
  point P8 (16, 10)
  dimension "d153" = 5
  dimension "d154" = 5
  dimension "d155" = 4
  dimension "d156" = 5
  dimension "d157" = 5
  dimension "d158" = 5
  dimension "d159" = 5
  dimension "d160" = 15
  constraints: 8 midpoint, 6 equal length, 6 horizontal, 5 horizontal alignment, 5 vertical alignment, 12 other
  measures "d153" distance of L0.start L0.end
  measures "d154" distance of L2.end L0.start
  measures "d155" distance of point (31, 41.5) A1.centre
  measures "d156" distance of L23.end L20.end
  measures "d157" distance of L23.start L23.end
  measures "d158" distance of L27.end L24.end
  measures "d159" distance of L27.start L27.end
  measures "d160" distance of A5.centre point (16, 25)
emboss "Emboss2" sketch "Sketch14" operation cut depth 1 direction (0, 0, 1)